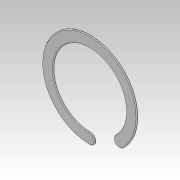
# Autodesk Inventor part: LogoCoverThin
Saved by Autodesk Inventor 2020 (Build 240168000, 168)
## iProperties
Created: 2022-08-30
Part Number: LogoCoverThin
Material: Generic
Document SubType Name: Modeling
Designer: DDeGo
Density: 1 g/cm^3
Appearance: Default
Author: DDeGo
Autodesk Inventor part; units mm, degrees
ref_plane "YZ Plane" through (0, 0, 0) normal (1, 0, 0) x (0, 1, 0)
ref_plane "XZ Plane" through (0, 0, 0) normal (0, 1, 0) x (-1, 0, 0)
ref_plane "XY Plane" through (0, 0, 0) normal (0, 0, 1) x (1, 0, 0)
sketch "Block1" plane through (0, 0, 0) normal (0, 0, 1) x (1, 0, 0)
  circle A0 centre (250, 0) radius 40 construction
  arc A1 (284, 0) -> (274.0416, -24.0416) centre (250, 0) ccw construction
  circle A2 centre (250, 0) radius 10.05 construction
  arc A3 (276, 0) -> (268.3848, -18.3848) centre (250, 0) ccw construction
  circle A4 centre (280, 0) radius 1.6 construction
  arc A5 (276, 0) -> (284, 0) centre (280, 0) ccw construction
  circle A6 centre (271.2132, -21.2132) radius 1.6 construction
  arc A7 (274.0416, -24.0416) -> (268.3848, -18.3848) centre (271.2132, -21.2132) ccw construction
  point P0 (269.205, -7.955)
  dimension "d0" = 8
  measures "d0" diameter of A5
sketch "Sketch1" plane through (0, 0, 0) normal (0, 0, 1) x (1, 0, 0)
  arc A0 (18.4908, -18.4908) -> (0, -26.15) centre (0, 0) ccw
  arc A1 (23.9356, -23.9356) -> (0, -33.85) centre (0, 0) ccw
  arc A2 (0, -33.85) -> (0, -26.15) centre (0, -30) ccw
  circle A3 centre (0, -30) radius 2.9
  arc A4 (18.4908, -18.4908) -> (23.9356, -23.9356) centre (21.2132, -21.2132) ccw
  circle A5 centre (21.2132, -21.2132) radius 2.9
  circle A6 centre (30, 0) radius 2.9
  circle A7 centre (21.2132, 21.2132) radius 2.9
  circle A8 centre (0, 30) radius 2.9
  circle A9 centre (-21.2132, 21.2132) radius 2.9
  circle A10 centre (-30, 0) radius 2.9
  circle A11 centre (-21.2132, -21.2132) radius 2.9
  point P0 (0, 0)
  point P1 (0, 0)
  dimension "d1" = 0.15
  dimension "d2" = 5.8
  dimension "d5" = 360
  constraints: 12 centre point, 8 point on circle, 3 coincident, 3 tangent, 22 other
  measures "d2" diameter of A3
extrude "Extrusion1" add sketch "Sketch1" along normal blind 0.2
sketch "Sketch2" plane through (0, 0, 0.2) normal (0, 0, 1) x (1, 0, 0)
  arc A0 (23.9356, -23.9356) -> (0, -33.85) centre (0, 0) ccw projected
  arc A1 (0, -33.85) -> (0, -26.15) centre (0, -30) ccw projected
  arc A2 (18.4908, -18.4908) -> (0, -26.15) centre (0, 0) ccw projected
  arc A3 (18.4908, -18.4908) -> (23.9356, -23.9356) centre (21.2132, -21.2132) ccw projected
  circle A4 centre (0, 30) radius 2.9 projected
  circle A5 centre (30, 0) radius 2.9 projected
  circle A6 centre (21.2132, -21.2132) radius 2.9 projected
  circle A7 centre (-30, 0) radius 2.9 projected
  circle A8 centre (-21.2132, -21.2132) radius 2.9 projected
  circle A9 centre (-21.2132, 21.2132) radius 2.9 projected
  circle A10 centre (21.2132, 21.2132) radius 2.9 projected
  circle A11 centre (0, -30) radius 2.9 projected
  point P0 (0, 0)
extrude "Extrusion2" add sketch "Sketch2" along normal blind 0.6 contours A3 A2 A1 A0 | A4 | A5 | A6 | A7 | A8 | A9 | A10 | A11
fillet "Fillet1" radius 0.5 4 edges at (3.85, -30, 0.8) (-10.0072, 24.1594, 0.8) (18.4908, -23.9356, 0.8) (-12.9538, 31.2733, 0.8)
sketch "Sketch3" plane through (0, 0, 0) normal (0, 0, -1) x (-1, 0, 0)
  circle A0 centre (0, -30) radius 2.9 projected
  circle A1 centre (-21.2132, -21.2132) radius 2.9 projected
  circle A2 centre (-30, 0) radius 2.9 projected
  circle A3 centre (-21.2132, 21.2132) radius 2.9 projected
  circle A4 centre (0, 30) radius 2.9 projected
  circle A5 centre (21.2132, 21.2132) radius 2.9 projected
  circle A6 centre (30, 0) radius 2.9 projected
  circle A7 centre (21.2132, -21.2132) radius 2.9 projected
  point P0 (0, 0)
extrude "Extrusion3" add sketch "Sketch3" against normal up to surface (0.2 mm away)
body "Solid1"
